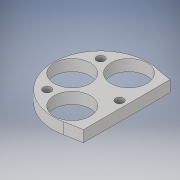
# Autodesk Inventor part: 000.403 -  Прижим подшипников
Saved by Autodesk Inventor 2019 (Build 230136000, 136)
## iProperties
Created: 2020-03-23
Part Number: 000.403 -  Прижим подшипников
Material: Типовые
Document SubType Name: Modeling
Designer: Петров Иван
Density: 1 g/cm^3
Appearance: По умолчанию
Author: Петров Иван
Autodesk Inventor part; units mm, degrees
ref_plane "YZ Plane" through (0, 0, 0) normal (1, 0, 0) x (0, 1, 0)
ref_plane "XZ Plane" through (0, 0, 0) normal (0, 1, 0) x (-1, 0, 0)
ref_plane "XY Plane" through (0, 0, 0) normal (0, 0, 1) x (1, 0, 0)
sketch "Эскиз1" plane through (0, 0, 0) normal (0, 1, 0) x (-1, 0, 0)
  circle A0 centre (15.0247, -0.005) radius 9.5
  circle A1 centre (0.0247, 14.995) radius 9.5
  circle A2 centre (0.0247, -15.005) radius 9.5
  arc A3 (-4.923, -24.5094) -> (-4.9258, 24.5) centre (0.0275, -0.0044) ccw
  arc A4 (-13.7779, 22.8932) -> (-4.9258, 24.5) centre (-49.9753, 247.495) ccw
  line L0 (-13.7779, 22.8932) -> (-13.7779, -22.9031)
  arc A5 (-4.923, -24.5094) -> (-4.9258, 24.5) centre (0.0275, -0.0044) ccw
  circle A6 centre (15.0247, -0.005) radius 9.5
  circle A7 centre (0.0247, 14.995) radius 9.5
  circle A8 centre (0.0247, -15.005) radius 9.5
  arc A9 (-4.923, -24.5094) -> (-4.9258, 24.5) centre (0.0275, -0.0044) ccw
  arc A10 (-13.7779, 22.8932) -> (-4.9258, 24.5) centre (-49.9753, 247.495) ccw
  arc A11 (-4.923, -24.5094) -> (-13.7779, -22.9031) centre (-49.9479, -247.5094) ccw
  line L1 (-13.7779, 22.8932) -> (-13.7779, -22.9031)
  arc A12 (-4.923, -24.5094) -> (-4.9258, 24.5) centre (0.0275, -0.0044) ccw
  point P0 (0, 0)
  constraints: 17 point on circle, 13 centre point, 4 end point, 2 coincident, 2 concentric, 2 vertical
extrude "Выдавливание1" add sketch "Эскиз1" along normal blind 6
sketch "Эскиз2" plane through (0, 6, 0) normal (0, 1, 0) x (1, 0, 0)
  line L0 (0, 0) -> (10, 0)
  circle A0 centre (10, 0) radius 2.1
  line L1 (0, 0) -> (-14.1421, -14.1421)
  line L2 (0, 0) -> (20, 0) construction
  line L3 (0, 0) -> (-14.1421, 14.1421)
  circle A1 centre (-14.1421, -14.1421) radius 2.1
  circle A2 centre (-14.1421, 14.1421) radius 2.1
  dimension "d2" = 10
  dimension "d3" = 4.2
  dimension "d4" = 20
  dimension "d5" = 135
  dimension "d6" = 20
  dimension "d7" = 90
  dimension "d8" = 4.2
  dimension "d9" = 4.2
  constraints: 8 end point, 3 centre point, 3 coincident, 2 horizontal, 1 equal length
  measures "d2" distance of L0.start L0.end
  measures "d3" diameter of A0
  measures "d4" distance of L0.start L1.end
  measures "d5" angle of L1 L2
  measures "d6" distance of L0.start L3.end
  measures "d7" angle of L1 L3
  measures "d8" diameter of A1
  measures "d9" diameter of A2
extrude "Выдавливание2" cut sketch "Эскиз2" against normal blind 15.25
equation "\"d3\" = d9"
equation "\"d8\" = d9"
